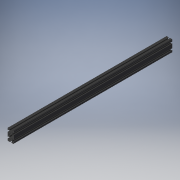
# Autodesk Inventor part: 30-3060-825-CL
Saved by Autodesk Inventor 2019 (Build 230136000, 136)
## iProperties
Created: 2023-03-27
Part Number: 30-3060-825-CL
Material: Generic
Catalog Web Link: www.cadenas.de
Description: 30-3060, 30-3060-Black-T-Slotted Profile - 30 Series
Vendor: 8020
Document SubType Name: Modeling
Designer: psAdmin
Manufacturer: 8020
Mass: 479.813 g
Surface Area: 4650.68 cm^2
Volume: 479.813 cm^3
Density: 1 g/cm^3
Appearance: PSOLRGB-191-191-191
Category: PARTsolutions
Company: 8020
Title: 30-3060-825
Author: Cadenas PARTsolutions
Comments: T-Slotted Profile - 30 Series
PSOL_IDENT_0: {$CADENAS_DATA/23d-libs/8020/metric/profiles/30_series/30_3060.prj},190 {VTYP=3D},{NB=30-3060-825-CL
PSOL_IDENT_1: },{LINA=30-3060-825},{NN=30-3060, 30-3060-Black},{DATE=31.07.2020 09:21:33},{GEOMDATE=01.11.2018 18:
PSOL_IDENT_2: 32:00},{VERSION=},{LINEID=10},{WBVAR=FIN,LS,L},{WBNUMERIC=L}  {NB=30-3060-825-CL},{LINA=30-3060-825}
PSOL_IDENT_3: ,{KT=DUMMY},{PN=30-3060-825},{PN1=30-3060},{FIN=CA},{LS=-CL},{L=825.00},{SERIES=30-3060},{MAT=6105-T
PSOL_IDENT_4: 5 Aluminum},{W=1.5060},{LALG=[25:6000/0.05]},{MIX=19.5737},{MIY=5.3856},{EA=6.4932},{COLOR=.75,.75,.
PSOL_IDENT_5: 75}
NB: 30-3060-825-CL
NN: 30-3060, 30-3060-Black
NT: T-Slotted Profile - 30 Series
NBSYN: $PN.$LS.
LINA: 30-3060-825
CATALOG: 80/20
PN: 30-3060-825
FIN: Clear Anodize
LS: Custom Length
L: 825
SERIES: 30-3060
MAT: 6105-T5 Aluminum
W: 1.5060
MIX: 19.5737
MIY: 5.3856
EA: 6.4932
SUPPLIER: 8020
ARTICLENO: 30-3060-825-CL
BOMINFO: 30-3060-825
CREATOR: CADENAS GmbH
Autodesk Inventor part; units mm, degrees
ref_plane "YZ Plane" through (0, 0, 0) normal (1, 0, 0) x (0, 1, 0)
ref_plane "XZ Plane" through (0, 0, 0) normal (0, 1, 0) x (-1, 0, 0)
ref_plane "XY Plane" through (0, 0, 0) normal (0, 0, 1) x (1, 0, 0)
sketch "Sketch_1" plane through (0, 0, 0) normal (0, 0, 1) x (1, 0, 0)
  arc A0 (-15, -13) -> (-13, -15) centre (-13, -13) ccw
  line L0 (-13, -15) -> (-4.508, -15)
  arc A1 (-4.508, -15) -> (-4, -14.492) centre (-4.508, -14.492) ccw
  line L1 (-4, -14.492) -> (-4, -13.251)
  arc A2 (-4, -13.251) -> (-4.508, -12.743) centre (-4.508, -13.251) ccw
  line L2 (-4.508, -12.743) -> (-7.742, -12.743)
  arc A3 (-8.25, -12.235) -> (-7.742, -12.743) centre (-7.742, -12.235) ccw
  line L3 (-8.25, -12.235) -> (-8.25, -10.2642)
  arc A4 (-8.1012, -9.905) -> (-8.25, -10.2642) centre (-7.742, -10.2642) ccw
  line L4 (-8.1012, -9.905) -> (-4.1795, -5.9833)
  arc A5 (-3.8203, -5.8345) -> (-4.1795, -5.9833) centre (-3.8203, -6.3425) ccw
  line L5 (-3.8203, -5.8345) -> (-0.949, -5.8345)
  line L6 (-0.949, -5.8345) -> (0, -5.325)
  line L7 (0, -5.325) -> (0.949, -5.8345)
  line L8 (0.949, -5.8345) -> (3.8216, -5.8345)
  arc A6 (4.1808, -5.9833) -> (3.8216, -5.8345) centre (3.8216, -6.3425) ccw
  line L9 (4.1808, -5.9833) -> (8.1012, -9.9037)
  arc A7 (8.25, -10.2629) -> (8.1012, -9.9037) centre (7.742, -10.2629) ccw
  line L10 (8.25, -10.2629) -> (8.25, -12.235)
  arc A8 (7.742, -12.743) -> (8.25, -12.235) centre (7.742, -12.235) ccw
  line L11 (7.742, -12.743) -> (4.508, -12.743)
  arc A9 (4.508, -12.743) -> (4, -13.251) centre (4.508, -13.251) ccw
  line L12 (4, -13.251) -> (4, -14.492)
  arc A10 (4, -14.492) -> (4.508, -15) centre (4.508, -14.492) ccw
  line L13 (4.508, -15) -> (13, -15)
  arc A11 (13, -15) -> (15, -13) centre (13, -13) ccw
  line L14 (15, -13) -> (15, -4.508)
  arc A12 (15, -4.508) -> (14.492, -4) centre (14.492, -4.508) ccw
  line L15 (14.492, -4) -> (13.251, -4)
  arc A13 (13.251, -4) -> (12.743, -4.508) centre (13.251, -4.508) ccw
  line L16 (12.743, -4.508) -> (12.743, -7.742)
  arc A14 (12.235, -8.25) -> (12.743, -7.742) centre (12.235, -7.742) ccw
  line L17 (12.235, -8.25) -> (10.2642, -8.25)
  arc A15 (9.905, -8.1012) -> (10.2642, -8.25) centre (10.2642, -7.742) ccw
  line L18 (9.905, -8.1012) -> (5.9833, -4.1795)
  arc A16 (5.8345, -3.8203) -> (5.9833, -4.1795) centre (6.3425, -3.8203) ccw
  line L19 (5.8345, -3.8203) -> (5.8345, -0.949)
  line L20 (5.8345, -0.949) -> (5.325, 0)
  line L21 (5.325, 0) -> (5.8345, 0.949)
  line L22 (5.8345, 0.949) -> (5.8345, 3.8216)
  arc A17 (5.9833, 4.1808) -> (5.8345, 3.8216) centre (6.3425, 3.8216) ccw
  line L23 (5.9833, 4.1808) -> (9.9037, 8.1012)
  arc A18 (10.2629, 8.25) -> (9.9037, 8.1012) centre (10.2629, 7.742) ccw
  line L24 (10.2629, 8.25) -> (12.235, 8.25)
  arc A19 (12.743, 7.742) -> (12.235, 8.25) centre (12.235, 7.742) ccw
  line L25 (12.743, 7.742) -> (12.743, 4.508)
  arc A20 (12.743, 4.508) -> (13.251, 4) centre (13.251, 4.508) ccw
  line L26 (13.251, 4) -> (14.492, 4)
  arc A21 (14.492, 4) -> (15, 4.508) centre (14.492, 4.508) ccw
  line L27 (15, 4.508) -> (15, 25.492)
  arc A22 (15, 25.492) -> (14.492, 26) centre (14.492, 25.492) ccw
  line L28 (14.492, 26) -> (13.251, 26)
  arc A23 (13.251, 26) -> (12.743, 25.492) centre (13.251, 25.492) ccw
  line L29 (12.743, 25.492) -> (12.743, 22.258)
  arc A24 (12.235, 21.75) -> (12.743, 22.258) centre (12.235, 22.258) ccw
  line L30 (12.235, 21.75) -> (10.2629, 21.75)
  arc A25 (9.9037, 21.8988) -> (10.2629, 21.75) centre (10.2629, 22.258) ccw
  line L31 (9.9037, 21.8988) -> (5.9833, 25.8192)
  arc A26 (5.8345, 26.1784) -> (5.9833, 25.8192) centre (6.3425, 26.1784) ccw
  line L32 (5.8345, 26.1784) -> (5.8345, 29.051)
  line L33 (5.8345, 29.051) -> (5.325, 30)
  line L34 (5.325, 30) -> (5.8345, 30.949)
  line L35 (5.8345, 30.949) -> (5.8345, 33.8203)
  arc A27 (5.9833, 34.1795) -> (5.8345, 33.8203) centre (6.3425, 33.8203) ccw
  line L36 (5.9833, 34.1795) -> (9.905, 38.1012)
  arc A28 (10.2642, 38.25) -> (9.905, 38.1012) centre (10.2642, 37.742) ccw
  line L37 (10.2642, 38.25) -> (12.235, 38.25)
  arc A29 (12.743, 37.742) -> (12.235, 38.25) centre (12.235, 37.742) ccw
  line L38 (12.743, 37.742) -> (12.743, 34.508)
  arc A30 (12.743, 34.508) -> (13.251, 34) centre (13.251, 34.508) ccw
  line L39 (13.251, 34) -> (14.492, 34)
  arc A31 (14.492, 34) -> (15, 34.508) centre (14.492, 34.508) ccw
  line L40 (15, 34.508) -> (15, 43)
  arc A32 (15, 43) -> (13, 45) centre (13, 43) ccw
  line L41 (13, 45) -> (4.508, 45)
  arc A33 (4.508, 45) -> (4, 44.492) centre (4.508, 44.492) ccw
  line L42 (4, 44.492) -> (4, 43.251)
  arc A34 (4, 43.251) -> (4.508, 42.743) centre (4.508, 43.251) ccw
  line L43 (4.508, 42.743) -> (7.742, 42.743)
  arc A35 (8.25, 42.235) -> (7.742, 42.743) centre (7.742, 42.235) ccw
  line L44 (8.25, 42.235) -> (8.25, 40.2629)
  arc A36 (8.1012, 39.9037) -> (8.25, 40.2629) centre (7.742, 40.2629) ccw
  line L45 (8.1012, 39.9037) -> (4.1808, 35.9833)
  arc A37 (3.8216, 35.8345) -> (4.1808, 35.9833) centre (3.8216, 36.3425) ccw
  line L46 (3.8216, 35.8345) -> (0.949, 35.8345)
  line L47 (0.949, 35.8345) -> (0, 35.325)
  line L48 (0, 35.325) -> (-0.949, 35.8345)
  line L49 (-0.949, 35.8345) -> (-3.8203, 35.8345)
  arc A38 (-4.1795, 35.9833) -> (-3.8203, 35.8345) centre (-3.8203, 36.3425) ccw
  line L50 (-4.1795, 35.9833) -> (-8.1012, 39.905)
  arc A39 (-8.25, 40.2642) -> (-8.1012, 39.905) centre (-7.742, 40.2642) ccw
  line L51 (-8.25, 40.2642) -> (-8.25, 42.235)
  arc A40 (-7.742, 42.743) -> (-8.25, 42.235) centre (-7.742, 42.235) ccw
  line L52 (-7.742, 42.743) -> (-4.508, 42.743)
  arc A41 (-4.508, 42.743) -> (-4, 43.251) centre (-4.508, 43.251) ccw
  line L53 (-4, 43.251) -> (-4, 44.492)
  arc A42 (-4, 44.492) -> (-4.508, 45) centre (-4.508, 44.492) ccw
  line L54 (-4.508, 45) -> (-13, 45)
  arc A43 (-13, 45) -> (-15, 43) centre (-13, 43) ccw
  line L55 (-15, 43) -> (-15, 34.508)
  arc A44 (-15, 34.508) -> (-14.492, 34) centre (-14.492, 34.508) ccw
  line L56 (-14.492, 34) -> (-13.251, 34)
  arc A45 (-13.251, 34) -> (-12.743, 34.508) centre (-13.251, 34.508) ccw
  line L57 (-12.743, 34.508) -> (-12.743, 37.742)
  arc A46 (-12.235, 38.25) -> (-12.743, 37.742) centre (-12.235, 37.742) ccw
  line L58 (-12.235, 38.25) -> (-10.2629, 38.25)
  arc A47 (-9.9037, 38.1012) -> (-10.2629, 38.25) centre (-10.2629, 37.742) ccw
  line L59 (-9.9037, 38.1012) -> (-5.9833, 34.1808)
  arc A48 (-5.8345, 33.8216) -> (-5.9833, 34.1808) centre (-6.3425, 33.8216) ccw
  line L60 (-5.8345, 33.8216) -> (-5.8345, 30.949)
  line L61 (-5.8345, 30.949) -> (-5.325, 30)
  line L62 (-5.325, 30) -> (-5.8345, 29.051)
  line L63 (-5.8345, 29.051) -> (-5.8345, 26.1797)
  arc A49 (-5.9833, 25.8205) -> (-5.8345, 26.1797) centre (-6.3425, 26.1797) ccw
  line L64 (-5.9833, 25.8205) -> (-9.905, 21.8988)
  arc A50 (-10.2642, 21.75) -> (-9.905, 21.8988) centre (-10.2642, 22.258) ccw
  line L65 (-10.2642, 21.75) -> (-12.235, 21.75)
  arc A51 (-12.743, 22.258) -> (-12.235, 21.75) centre (-12.235, 22.258) ccw
  line L66 (-12.743, 22.258) -> (-12.743, 25.492)
  arc A52 (-12.743, 25.492) -> (-13.251, 26) centre (-13.251, 25.492) ccw
  line L67 (-13.251, 26) -> (-14.492, 26)
  arc A53 (-14.492, 26) -> (-15, 25.492) centre (-14.492, 25.492) ccw
  line L68 (-15, 25.492) -> (-15, 4.508)
  arc A54 (-15, 4.508) -> (-14.492, 4) centre (-14.492, 4.508) ccw
  line L69 (-14.492, 4) -> (-13.251, 4)
  arc A55 (-13.251, 4) -> (-12.743, 4.508) centre (-13.251, 4.508) ccw
  line L70 (-12.743, 4.508) -> (-12.743, 7.742)
  arc A56 (-12.235, 8.25) -> (-12.743, 7.742) centre (-12.235, 7.742) ccw
  line L71 (-12.235, 8.25) -> (-10.2642, 8.25)
  arc A57 (-9.905, 8.1012) -> (-10.2642, 8.25) centre (-10.2642, 7.742) ccw
  line L72 (-9.905, 8.1012) -> (-5.9833, 4.1795)
  arc A58 (-5.8345, 3.8203) -> (-5.9833, 4.1795) centre (-6.3425, 3.8203) ccw
  line L73 (-5.8345, 3.8203) -> (-5.8345, 0.949)
  line L74 (-5.8345, 0.949) -> (-5.325, 0)
  line L75 (-5.325, 0) -> (-5.8345, -0.949)
  line L76 (-5.8345, -0.949) -> (-5.8345, -3.8216)
  arc A59 (-5.9833, -4.1808) -> (-5.8345, -3.8216) centre (-6.3425, -3.8216) ccw
  line L77 (-5.9833, -4.1808) -> (-9.9037, -8.1012)
  arc A60 (-10.2629, -8.25) -> (-9.9037, -8.1012) centre (-10.2629, -7.742) ccw
  line L78 (-10.2629, -8.25) -> (-12.235, -8.25)
  arc A61 (-12.743, -7.742) -> (-12.235, -8.25) centre (-12.235, -7.742) ccw
  line L79 (-12.743, -7.742) -> (-12.743, -4.508)
  arc A62 (-12.743, -4.508) -> (-13.251, -4) centre (-13.251, -4.508) ccw
  line L80 (-13.251, -4) -> (-14.492, -4)
  arc A63 (-14.492, -4) -> (-15, -4.508) centre (-14.492, -4.508) ccw
  line L81 (-15, -4.508) -> (-15, -13)
  arc A64 (9.5, -13.319) -> (9.881, -13.7) centre (9.881, -13.319) ccw
  line L82 (9.881, -13.7) -> (12.7, -13.7)
  arc A65 (12.7, -13.7) -> (13.7, -12.7) centre (12.7, -12.7) ccw
  line L83 (13.7, -12.7) -> (13.7, -9.881)
  arc A66 (13.7, -9.881) -> (13.319, -9.5) centre (13.319, -9.881) ccw
  line L84 (13.319, -9.5) -> (9.881, -9.5)
  arc A67 (9.881, -9.5) -> (9.5, -9.881) centre (9.881, -9.881) ccw
  line L85 (9.5, -9.881) -> (9.5, -13.319)
  line L86 (9.5, 43.319) -> (9.5, 39.881)
  arc A68 (9.5, 39.881) -> (9.881, 39.5) centre (9.881, 39.881) ccw
  line L87 (9.881, 39.5) -> (13.319, 39.5)
  arc A69 (13.319, 39.5) -> (13.7, 39.881) centre (13.319, 39.881) ccw
  line L88 (13.7, 39.881) -> (13.7, 42.7)
  arc A70 (13.7, 42.7) -> (12.7, 43.7) centre (12.7, 42.7) ccw
  line L89 (12.7, 43.7) -> (9.881, 43.7)
  arc A71 (9.881, 43.7) -> (9.5, 43.319) centre (9.881, 43.319) ccw
  arc A72 (-4.0107, -2.5139) -> (-2.5139, -4.0107) centre (-3.142, -3.142) ccw
  line L90 (-2.5139, -4.0107) -> (-1.3138, -3.0544)
  arc A73 (-1.3138, -3.0544) -> (1.3138, -3.0544) centre (0, 0) ccw
  line L91 (1.3138, -3.0544) -> (2.5139, -4.0107)
  arc A74 (2.5139, -4.0107) -> (4.0107, -2.5139) centre (3.142, -3.142) ccw
  line L92 (4.0107, -2.5139) -> (3.0544, -1.3138)
  arc A75 (3.0544, -1.3138) -> (3.0544, 1.3138) centre (0, 0) ccw
  line L93 (3.0544, 1.3138) -> (4.0107, 2.5139)
  arc A76 (4.0107, 2.5139) -> (2.5139, 4.0107) centre (3.142, 3.142) ccw
  line L94 (2.5139, 4.0107) -> (1.3138, 3.0544)
  arc A77 (1.3138, 3.0544) -> (-1.3138, 3.0544) centre (0, 0) ccw
  line L95 (-1.3138, 3.0544) -> (-2.5139, 4.0107)
  arc A78 (-2.5139, 4.0107) -> (-4.0107, 2.5139) centre (-3.142, 3.142) ccw
  line L96 (-4.0107, 2.5139) -> (-3.0544, 1.3138)
  arc A79 (-3.0544, 1.3138) -> (-3.0544, -1.3138) centre (0, 0) ccw
  line L97 (-3.0544, -1.3138) -> (-4.0107, -2.5139)
  arc A80 (-2.5139, 34.0107) -> (-4.0107, 32.5139) centre (-3.142, 33.142) ccw
  line L98 (-4.0107, 32.5139) -> (-3.0544, 31.3138)
  arc A81 (-3.0544, 31.3138) -> (-3.0544, 28.6862) centre (0, 30) ccw
  line L99 (-3.0544, 28.6862) -> (-4.0107, 27.4861)
  arc A82 (-4.0107, 27.4861) -> (-2.5139, 25.9893) centre (-3.142, 26.858) ccw
  line L100 (-2.5139, 25.9893) -> (-1.3138, 26.9456)
  arc A83 (-1.3138, 26.9456) -> (1.3138, 26.9456) centre (0, 30) ccw
  line L101 (1.3138, 26.9456) -> (2.5139, 25.9893)
  arc A84 (2.5139, 25.9893) -> (4.0107, 27.4861) centre (3.142, 26.858) ccw
  line L102 (4.0107, 27.4861) -> (3.0544, 28.6862)
  arc A85 (3.0544, 28.6862) -> (3.0544, 31.3138) centre (0, 30) ccw
  line L103 (3.0544, 31.3138) -> (4.0107, 32.5139)
  arc A86 (4.0107, 32.5139) -> (2.5139, 34.0107) centre (3.142, 33.142) ccw
  line L104 (2.5139, 34.0107) -> (1.3138, 33.0544)
  arc A87 (1.3138, 33.0544) -> (-1.3138, 33.0544) centre (0, 30) ccw
  line L105 (-1.3138, 33.0544) -> (-2.5139, 34.0107)
  line L106 (-12.8, 19.05) -> (-12.8, 10.95)
  arc A88 (-12.8, 10.95) -> (-12.3, 10.45) centre (-12.3, 10.95) ccw
  line L107 (-12.3, 10.45) -> (-9.2688, 10.45)
  arc A89 (-8.2082, 10.0107) -> (-9.2688, 10.45) centre (-9.2688, 8.95) ccw
  line L108 (-8.2082, 10.0107) -> (-4.1808, 5.9833)
  arc A90 (-4.1808, 5.9833) -> (-3.8216, 5.8345) centre (-3.8216, 6.3425) ccw
  line L109 (-3.8216, 5.8345) -> (-0.949, 5.8345)
  line L110 (-0.949, 5.8345) -> (0, 5.325)
  line L111 (0, 5.325) -> (0.949, 5.8345)
  line L112 (0.949, 5.8345) -> (3.8203, 5.8345)
  arc A91 (3.8203, 5.8345) -> (4.1795, 5.9833) centre (3.8203, 6.3425) ccw
  line L113 (4.1795, 5.9833) -> (8.2069, 10.0107)
  arc A92 (9.2676, 10.45) -> (8.2069, 10.0107) centre (9.2676, 8.95) ccw
  line L114 (9.2676, 10.45) -> (12.3, 10.45)
  arc A93 (12.3, 10.45) -> (12.8, 10.95) centre (12.3, 10.95) ccw
  line L115 (12.8, 10.95) -> (12.8, 19.05)
  arc A94 (12.8, 19.05) -> (12.3, 19.55) centre (12.3, 19.05) ccw
  line L116 (12.3, 19.55) -> (9.2676, 19.55)
  arc A95 (8.2069, 19.9893) -> (9.2676, 19.55) centre (9.2676, 21.05) ccw
  line L117 (8.2069, 19.9893) -> (4.1795, 24.0167)
  arc A96 (4.1795, 24.0167) -> (3.8203, 24.1655) centre (3.8203, 23.6575) ccw
  line L118 (3.8203, 24.1655) -> (0.949, 24.1655)
  line L119 (0.949, 24.1655) -> (0, 24.675)
  line L120 (0, 24.675) -> (-0.949, 24.1655)
  line L121 (-0.949, 24.1655) -> (-3.8216, 24.1655)
  arc A97 (-3.8216, 24.1655) -> (-4.1808, 24.0167) centre (-3.8216, 23.6575) ccw
  line L122 (-4.1808, 24.0167) -> (-8.2082, 19.9893)
  arc A98 (-9.2688, 19.55) -> (-8.2082, 19.9893) centre (-9.2688, 21.05) ccw
  line L123 (-9.2688, 19.55) -> (-12.3, 19.55)
  arc A99 (-12.3, 19.55) -> (-12.8, 19.05) centre (-12.3, 19.05) ccw
  arc A100 (-13.7, -12.7) -> (-12.7, -13.7) centre (-12.7, -12.7) ccw
  line L124 (-12.7, -13.7) -> (-9.881, -13.7)
  arc A101 (-9.881, -13.7) -> (-9.5, -13.319) centre (-9.881, -13.319) ccw
  line L125 (-9.5, -13.319) -> (-9.5, -9.881)
  arc A102 (-9.5, -9.881) -> (-9.881, -9.5) centre (-9.881, -9.881) ccw
  line L126 (-9.881, -9.5) -> (-13.319, -9.5)
  arc A103 (-13.319, -9.5) -> (-13.7, -9.881) centre (-13.319, -9.881) ccw
  line L127 (-13.7, -9.881) -> (-13.7, -12.7)
  line L128 (-13.7, 42.7) -> (-13.7, 39.881)
  arc A104 (-13.7, 39.881) -> (-13.319, 39.5) centre (-13.319, 39.881) ccw
  line L129 (-13.319, 39.5) -> (-9.881, 39.5)
  arc A105 (-9.881, 39.5) -> (-9.5, 39.881) centre (-9.881, 39.881) ccw
  line L130 (-9.5, 39.881) -> (-9.5, 43.319)
  arc A106 (-9.5, 43.319) -> (-9.881, 43.7) centre (-9.881, 43.319) ccw
  line L131 (-9.881, 43.7) -> (-12.7, 43.7)
  arc A107 (-12.7, 43.7) -> (-13.7, 42.7) centre (-12.7, 42.7) ccw
  constraints: 264 end point, 216 point on circle, 108 centre point
extrude "Extrusion1" add sketch "Sketch_1" against normal blind 825
body "Solid1"
